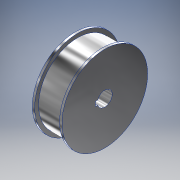
# Autodesk Inventor part: Puleggia minore
Saved by Autodesk Inventor 2018 (Build 220112000, 112)
## iProperties
Created: 2020-06-04
Part Number: Puleggia minore
Material: Alluminio 6061
Document SubType Name: Modeling
Designer: Francesco
Density: 2.7 g/cm^3
Appearance: Alluminio - Piatto
Mass: 597.839 g
Surface Area: 325.269 cm^2
Volume: 221.422 cm^3
Author: Francesco
Autodesk Inventor part; units mm, degrees
ref_plane "YZ Plane" through (0, 0, 0) normal (1, 0, 0) x (0, 1, 0)
ref_plane "XZ Plane" through (0, 0, 0) normal (0, 1, 0) x (-1, 0, 0)
ref_plane "XY Plane" through (0, 0, 0) normal (0, 0, 1) x (1, 0, 0)
sketch "Schizzo1" plane through (0, 0, 0) normal (0, 0, 1) x (1, 0, 0)
  line L0 (-16, 50) -> (16, 50)
  line L1 (-16, 50) -> (-16, 57)
  line L2 (-16, 57) -> (-19, 57)
  line L3 (-19, 57) -> (-19, 0)
  line L4 (16, 50) -> (16, 57)
  line L5 (16, 57) -> (19, 57)
  line L6 (19, 57) -> (19, 0)
  line L7 (-19, 0) -> (19, 0)
  point P0 (0, 0)
  point P1 (0, 0)
  dimension "d2" = 7
  dimension "d3" = 3
  dimension "d4" = 3
  dimension "d5" = 7
  dimension "d6" = 100
  dimension "d7" = 32
  dimension "d8" = 38
  constraints: 16 end point, 3 perpendicular, 2 coincident, 2 horizontal, 2 vertical, 1 horizontal alignment, 1 midpoint
  measures "d2" distance of L0.start L1.end
  measures "d3" distance of L1.end L2.end
  measures "d4" distance of L4.end L5.end
  measures "d5" distance between parallel lines of L0 L5
  measures "d6" diameter of L0 L7
  measures "d7" distance between parallel lines of L4 L1
  measures "d8" distance between parallel lines of L6 L3
revolve "Rivoluzione1" add sketch "Schizzo1" angle 360 about axis through (-19, 0, 0) along (1, 0, 0)
sketch "Schizzo3" plane through (19, 0, 0) normal (1, 0, 0) x (0, 0, -1)
  arc A0 (3, -9.0139) -> (-3, -9.0139) centre (0, 0) ccw projected
  line L0 (3, -12) -> (-3, -12) projected
  arc A1 (3, -9.0139) -> (-3, -9.0139) centre (0, 0) ccw
  line L1 (-3, -12) -> (3, -12)
  line L2 (3, -12) -> (3, -9.0139)
  line L3 (-3, -12) -> (-3, -9.0139)
  point P0 (0, 0)
  constraints: 6 end point, 2 equal length, 2 point on circle, 1 centre point, 1 coincident, 1 concentric, 1 vertical
extrude "Estrusione2" cut sketch "Schizzo3" against normal up to next
